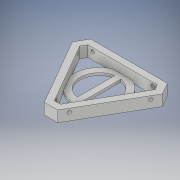
# Autodesk Inventor part: Stewart_Platform
Saved by Autodesk Inventor 2018.1 (Build 221171000, 171)
## iProperties
Created: 2017-11-13
Part Number: Stewart_Platform
Material: Generic
Document SubType Name: Modeling
Designer: sodie
Density: 1 g/cm^3
Appearance: Default
Author: sodie
Autodesk Inventor part; units mm, degrees
ref_plane "YZ Plane" through (0, 0, 0) normal (1, 0, 0) x (0, 1, 0)
ref_plane "XZ Plane" through (0, 0, 0) normal (0, 1, 0) x (-1, 0, 0)
ref_plane "XY Plane" through (0, 0, 0) normal (0, 0, 1) x (1, 0, 0)
sketch "Sketch1" plane through (0, 0, 0) normal (0, 1, 0) x (-1, 0, 0)
  circle A0 centre (0, 0) radius 50
  line L0 (35.3554, -35.3553) -> (42.8554, -35.3553) construction
  line L1 (48.2963, -12.941) -> (55.7963, -12.941) construction
  line L2 (12.9409, 48.2963) -> (20.4409, 48.2963) construction
  line L3 (-12.941, 48.2963) -> (-5.441, 48.2963) construction
  line L4 (-48.2963, -12.941) -> (-40.7963, -12.941) construction
  line L5 (-35.3553, -35.3553) -> (-27.8553, -35.3553) construction
  line L6 (45.3554, -35.3553) -> (53.2963, -21.6012)
  line L7 (-45.3554, -35.3553) -> (-53.2964, -21.6012)
  line L8 (-7.941, 56.9566) -> (7.9409, 56.9566)
  line L9 (7.9409, 56.9566) -> (53.2963, -21.6012)
  line L10 (-45.3554, -35.3553) -> (45.3554, -35.3553)
  line L11 (-53.2964, -21.6012) -> (-7.941, 56.9566)
  line L12 (44.636, -21.6012) -> (41.0252, -27.8553)
  line L13 (41.0252, -27.8553) -> (-41.0253, -27.8553)
  line L14 (-41.0253, -27.8553) -> (-44.6361, -21.6012)
  line L15 (-44.6361, -21.6012) -> (-3.6108, 49.4566)
  line L16 (-3.6108, 49.4566) -> (3.6108, 49.4566)
  line L17 (3.6108, 49.4566) -> (44.636, -21.6012)
  arc A1 (0, -27.8553) -> (0.0657, -27.8553) centre (0.0328, 0.0001) ccw
  circle A2 centre (0, 0) radius 22.5
  line L18 (3.6108, -27.8553) -> (-3.6108, -27.8553)
  line L19 (-3.6108, -27.8553) -> (-3.6108, 49.4566)
  line L20 (-3.6108, 49.4566) -> (3.6108, 49.4566)
  line L21 (3.6108, 49.4566) -> (3.6108, -27.8553)
  circle A3 centre (0, 0) radius 30
  point P0 (0, -27.8553)
  point P1 (0, -27.8553)
  point P2 (0, 49.4566)
  point P3 (0, 49.4566)
  dimension "d0" = 100
  dimension "d7" = 35.3553
  dimension "d9" = 12.941
  dimension "d10" = 48.2963
  dimension "d11" = 35.3553
  dimension "d12" = 35.3553
  dimension "d13" = 35.3554
  dimension "d17" = 12.941
  dimension "d18" = 48.2963
  dimension "d20" = 48.2963
  dimension "d21" = 12.9409
  dimension "d22" = 48.2963
  dimension "d23" = 12.941
  dimension "d99" = 7.5
  dimension "d133" = 2.5
  dimension "d134" = 15.8819
  dimension "d140" = 15.8819
  dimension "d143" = 15.8819
  dimension "d144" = 90.7107
  dimension "d145" = 90.7108
  dimension "d146" = 90.7107
  dimension "d147" = 35.3553
  dimension "d148" = 120
  dimension "d149" = 120
  dimension "d150" = 7.5
  dimension "d184" = 45
  dimension "d185" = 60
  constraints: 44 end point, 9 horizontal, 4 centre point, 4 midpoint, 4 point on circle, 2 coincident, 2 horizontal alignment, 2 parallel, 2 point on line, 1 perpendicular, 1 vertical alignment, 5 other
  measures "d0" diameter of A0
  measures "d7" horizontal distance of point (0, 0) L5.start
  measures "d9" vertical distance of point (0, 0) L4.start
  measures "d10" horizontal distance of point (0, 0) L4.start
  measures "d11" horizontal distance of point (0, 0) L5.start
  measures "d12" horizontal distance of point (0, 0) L0.start
  measures "d13" horizontal distance of point (0, 0) L0.start
  measures "d17" vertical distance of point (0, 0) L1.start
  measures "d18" horizontal distance of point (0, 0) L1.start
  measures "d20" vertical distance of L2.start point (0, 0)
  measures "d21" horizontal distance of point (0, 0) L2.start
  measures "d22" vertical distance of L3.start point (0, 0)
  measures "d23" horizontal distance of L3.start point (0, 0)
  measures "d99" distance of L0.start L0.end
  measures "d133" distance of L0.end L6.start
  measures "d134" distance of L6.start L6.end
  measures "d140" distance of L7.start L7.end
  measures "d143" distance of L8.start L8.end
  measures "d144" distance of L8.end L6.end
  measures "d145" distance of L7.start L6.start
  measures "d146" distance of L7.end L8.start
  measures "d147" distance from line of point (0, 0) L10
  measures "d148" angle of L10 L7
  measures "d149" angle of L7 L11
  measures "d150" distance between parallel lines of L9 L17
  measures "d184" diameter of A2
  measures "d185" diameter of A3
extrude "Extrusion5" add sketch "Sketch1" along normal blind 13 contours L9 A0 L10 L11 | A0 L11 L8 L9 | L9 L6 L10 A0 | A0 L10 L7 L11 | L17 A3 | A3 L13 | A3 L15
sketch "Sketch5" plane through (53.2964, 0, -21.6012) normal (0.866, 0, 0.5) x (0.5, 0, -0.866)
  circle A0 centre (-80.7107, 9) radius 2
  circle A1 centre (-10, 9) radius 2
  line L0 (-90.7107, 13) -> (0, 13) projected
  line L1 (-90.7107, 0) -> (-90.7107, 13) projected
  line L2 (0, 0) -> (0, 13) projected
  point P0 (-45.3554, 0)
  dimension "d155" = 4
  dimension "d156" = 4
  dimension "d157" = 4
  dimension "d158" = 10
  dimension "d159" = 10
  constraints: 2 centre point, 1 horizontal alignment
  measures "d155" diameter of A0
  measures "d156" diameter of A1
  measures "d157" distance from line of L0 A0.centre
  measures "d158" distance from line of L1 A0.centre
  measures "d159" distance from line of L2 A1.centre
sketch "Sketch6" plane through (-7.9409, 0, 56.9566) normal (-0.866, 0, 0.5) x (0.5, 0, 0.866)
  circle A0 centre (-80.7107, 9) radius 2
  circle A1 centre (-10, 9) radius 2
  line L0 (0, 0) -> (0, 13) projected
  line L1 (-90.7107, 13) -> (0, 13) projected
  line L2 (-90.7107, 0) -> (-90.7107, 13) projected
  point P0 (-45.3554, 0)
  dimension "d160" = 4
  dimension "d161" = 4
  dimension "d162" = 10
  dimension "d163" = 4
  dimension "d164" = 10
  constraints: 2 centre point, 1 horizontal alignment
  measures "d160" diameter of A0
  measures "d161" diameter of A1
  measures "d162" distance from line of L0 A1.centre
  measures "d163" distance from line of L1 A0.centre
  measures "d164" distance from line of L2 A0.centre
sketch "Sketch7" plane through (45.3554, 0, -35.3553) normal (0, 0, -1) x (-1, 0, 0)
  circle A0 centre (10, 9) radius 2
  circle A1 centre (80.7107, 9) radius 2
  line L0 (0, 13) -> (90.7107, 13) projected
  line L1 (0, 0) -> (0, 13) projected
  line L2 (90.7107, 0) -> (90.7107, 13) projected
  point P0 (45.3554, 0)
  dimension "d165" = 4
  dimension "d166" = 4
  dimension "d167" = 4
  dimension "d168" = 10
  dimension "d169" = 10
  constraints: 2 centre point, 1 horizontal alignment
  measures "d165" diameter of A0
  measures "d166" diameter of A1
  measures "d167" distance from line of L0 A0.centre
  measures "d168" distance from line of L1 A0.centre
  measures "d169" distance from line of L2 A1.centre
extrude "Extrusion6" cut sketch "Sketch5" against normal blind 7.5
extrude "Extrusion7" cut sketch "Sketch7" against normal blind 7.5
extrude "Extrusion8" cut sketch "Sketch6" against normal blind 7.5
extrude "Extrusion9" add sketch "Sketch1" along normal blind 3 contours A3 L13 L21 A2 L17 | L17 A3 | A3 L13 | L13 L19 A2 L21 | A3 L15 L19 A2 L13 | L21 A3 L19 L16 | L21 A2 L19 A3 | A2 L19 L21 | A3 L15
body "Solid4"
